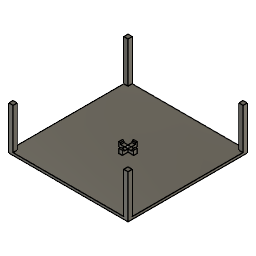
Desk (Autodesk Fusion 360 design; units mm, degrees)
part number: 2026-02-08-13-47-04-236
Autodesk Fusion 360 part; units mm, degrees
sketch "Sketch1" plane through (0, 0, 0) normal (0, 0, 1) x (1, 0, 0)
  line L0 (-44.8667, 47.2814) -> (95.1333, 47.2814)
  line L1 (95.1333, 47.2814) -> (95.1333, -92.7186)
  line L2 (95.1333, -92.7186) -> (-44.8667, -92.7186)
  line L3 (-44.8667, -92.7186) -> (-44.8667, 47.2814)
  dimension "d1" = 140
  dimension "d2" = 140
  constraint horizontal L0
  constraint vertical L1
  constraint horizontal L2
  constraint vertical L3
  measures "d1" distance of L0.start L0.end
  measures "d2" distance of L0.start L2.end
extrude "Extrude1" add sketch "Sketch1" along normal blind 3
sketch "Sketch2" plane through (0, 0, 3) normal (0, 0, 1) x (-1, 0, 0)
  line L0 (44.8667, 92.7186) -> (-95.1333, 92.7186)
  line L1 (-95.1333, 92.7186) -> (-95.1333, -47.2814)
  line L2 (-95.1333, -47.2814) -> (44.8667, -47.2814)
  line L3 (44.8667, -47.2814) -> (44.8667, 92.7186)
  line L4 (44.8667, -47.2814) -> (39.8667, -47.2814)
  line L5 (39.8667, -47.2814) -> (39.8667, -42.2814)
  line L6 (39.8667, -42.2814) -> (44.8667, -42.2814)
  line L7 (44.8667, -42.2814) -> (44.8667, -47.2814)
  line L8 (44.8667, 92.7186) -> (39.8667, 92.7186)
  line L9 (39.8667, 92.7186) -> (39.8667, 87.7186)
  line L10 (39.8667, 87.7186) -> (44.8667, 87.7186)
  line L11 (44.8667, 87.7186) -> (44.8667, 92.7186)
  line L12 (-95.1333, 92.7186) -> (-90.1333, 92.7186)
  line L13 (-90.1333, 92.7186) -> (-90.1333, 87.7186)
  line L14 (-90.1333, 87.7186) -> (-95.1333, 87.7186)
  line L15 (-95.1333, 87.7186) -> (-95.1333, 92.7186)
  line L16 (-95.1333, -47.2814) -> (-90.1333, -47.2814)
  line L17 (-90.1333, -47.2814) -> (-90.1333, -42.2814)
  line L18 (-90.1333, -42.2814) -> (-95.1333, -42.2814)
  line L19 (-95.1333, -42.2814) -> (-95.1333, -47.2814)
  dimension "d5" = 5
  dimension "d6" = 5
  dimension "d7" = 5
  dimension "d8" = 5
  dimension "d9" = 5
  dimension "d10" = 5
  dimension "d11" = 5
  dimension "d12" = 5
  constraint horizontal L4
  constraint vertical L5
  constraint horizontal L6
  constraint vertical L7
  constraint coincident L2.end L3.start
  constraint horizontal L8
  constraint vertical L9
  constraint horizontal L10
  constraint vertical L11
  constraint coincident L0.start L3.end
  constraint horizontal L12
  constraint vertical L13
  constraint horizontal L14
  constraint vertical L15
  constraint coincident L0.end L1.start
  constraint horizontal L16
  constraint vertical L17
  constraint horizontal L18
  constraint vertical L19
  constraint coincident L1.end L2.start
  measures "d5" distance of L2.end L4.end
  measures "d6" distance of L2.end L6.end
  measures "d7" distance of L0.start L8.end
  measures "d8" distance of L0.start L10.end
  measures "d9" distance of L0.end L12.end
  measures "d10" distance of L0.end L14.end
  measures "d11" distance of L1.end L16.end
  measures "d12" distance of L1.end L18.end
extrude "Extrude2" add sketch "Sketch2" along normal blind 48 contours L0 L3 L8 L9 L10 L11 | L0 L1 L12 L13 L14 L15 | L2 L3 L4 L5 L6 L7 | L1 L2 L16 L17 L18 L19
sketch "Sketch3" plane through (0, 0, 3) normal (0, 0, 1) x (-1, 0, 0)
  line L0 (-90.1333, 92.7186) -> (-90.1333, 87.7186)
  line L1 (-90.1333, 87.7186) -> (-95.1333, 87.7186)
  line L2 (-95.1333, 87.7186) -> (-95.1333, -42.2814)
  line L3 (-95.1333, -42.2814) -> (-90.1333, -42.2814)
  line L4 (-90.1333, -42.2814) -> (-90.1333, -47.2814)
  line L5 (-90.1333, -47.2814) -> (39.8667, -47.2814)
  line L6 (39.8667, -47.2814) -> (39.8667, -42.2814)
  line L7 (39.8667, -42.2814) -> (44.8667, -42.2814)
  line L8 (44.8667, -42.2814) -> (44.8667, 87.7186)
  line L9 (44.8667, 87.7186) -> (39.8667, 87.7186)
  line L10 (39.8667, 87.7186) -> (39.8667, 92.7186)
  line L11 (39.8667, 92.7186) -> (-90.1333, 92.7186)
  circle A0 centre (-25.1333, 22.7186) radius 2
  line L12 (-27.1333, 31.4686) -> (-23.1333, 31.4686)
  line L13 (-23.1333, 31.4686) -> (-23.1333, 13.9686)
  line L14 (-23.1333, 13.9686) -> (-27.1333, 13.9686)
  line L15 (-27.1333, 13.9686) -> (-27.1333, 31.4686)
  line L16 (-33.8833, 24.7186) -> (-16.3833, 24.7186)
  line L17 (-16.3833, 24.7186) -> (-16.3833, 20.7186)
  line L18 (-16.3833, 20.7186) -> (-33.8833, 20.7186)
  line L19 (-33.8833, 20.7186) -> (-33.8833, 24.7186)
  dimension "d15" = 4
  dimension "d16" = 70
  dimension "d17" = 70
  dimension "d18" = 4
  dimension "d19" = 17.5
  dimension "d20" = 8.75
  dimension "d21" = 2
  dimension "d22" = 17.5
  dimension "d23" = 4
  dimension "d24" = 2
  dimension "d25" = 8.75
  constraint horizontal L12
  constraint vertical L13
  constraint horizontal L14
  constraint vertical L15
  constraint horizontal L16
  constraint vertical L17
  constraint horizontal L18
  constraint vertical L19
  measures "d15" diameter of A0
  measures "d16" distance of L8 A0.centre
  measures "d17" distance of L11 A0.centre
  measures "d18" distance of L12.start L12.end
  measures "d19" distance of L12.start L14.end
  measures "d20" distance of A0.centre L12
  measures "d21" distance of A0.centre L15
  measures "d22" distance of L16.start L16.end
  measures "d23" distance of L16.start L18.end
  measures "d24" distance of A0.centre L18
  measures "d25" distance of A0.centre L19
extrude "Extrude3" add sketch "Sketch3" along normal blind 3.3 contours A0 L13 L18 | A0 L13 L16 | L13 L16 L17 L18 | A0 L15 L16 | L12 L13 L15 L16 | A0 L15 L18 | L13 L14 L15 L18 | L15 L16 L18 L19
sketch "Sketch4" plane through (0, 0, 6.3) normal (0, 0, 1) x (-1, 0, 0)
  circle A0 centre (-25.1333, 22.7186) radius 2
  line L0 (-33.8833, 20.7186) -> (-27.1333, 20.7186)
  line L1 (-27.1333, 20.7186) -> (-27.1333, 13.9686)
  line L2 (-27.1333, 13.9686) -> (-23.1333, 13.9686)
  line L3 (-23.1333, 13.9686) -> (-23.1333, 20.7186)
  line L4 (-23.1333, 20.7186) -> (-16.3833, 20.7186)
  line L5 (-16.3833, 20.7186) -> (-16.3833, 24.7186)
  line L6 (-16.3833, 24.7186) -> (-23.1333, 24.7186)
  line L7 (-23.1333, 24.7186) -> (-23.1333, 31.4686)
  line L8 (-23.1333, 31.4686) -> (-27.1333, 31.4686)
  line L9 (-27.1333, 31.4686) -> (-27.1333, 24.7186)
  line L10 (-27.1333, 24.7186) -> (-33.8833, 24.7186)
  line L11 (-33.8833, 24.7186) -> (-33.8833, 20.7186)
  line L12 (-27.1333, 31.4686) -> (-23.1333, 31.4686)
  line L13 (-23.1333, 31.4686) -> (-23.1333, 29.4686)
  line L14 (-23.1333, 29.4686) -> (-27.1333, 29.4686)
  line L15 (-27.1333, 29.4686) -> (-27.1333, 31.4686)
  line L16 (-16.3833, 24.7186) -> (-18.3833, 24.7186)
  line L17 (-18.3833, 24.7186) -> (-18.3833, 20.7186)
  line L18 (-18.3833, 20.7186) -> (-16.3833, 20.7186)
  line L19 (-16.3833, 20.7186) -> (-16.3833, 24.7186)
  line L20 (-23.1333, 13.9686) -> (-27.1333, 13.9686)
  line L21 (-27.1333, 13.9686) -> (-27.1333, 15.9686)
  line L22 (-27.1333, 15.9686) -> (-23.1333, 15.9686)
  line L23 (-23.1333, 15.9686) -> (-23.1333, 13.9686)
  line L24 (-33.8833, 24.7186) -> (-31.8833, 24.7186)
  line L25 (-31.8833, 24.7186) -> (-31.8833, 20.7186)
  line L26 (-31.8833, 20.7186) -> (-33.8833, 20.7186)
  line L27 (-33.8833, 20.7186) -> (-33.8833, 24.7186)
  dimension "d28" = 2
  dimension "d29" = 2
  dimension "d30" = 4
  dimension "d31" = 4
  dimension "d32" = 2
  dimension "d33" = 2
  dimension "d34" = 4
  dimension "d40" = 4
  constraint horizontal L12
  constraint vertical L13
  constraint horizontal L14
  constraint vertical L15
  constraint coincident L8.end L9.start
  constraint horizontal L16
  constraint vertical L17
  constraint horizontal L18
  constraint vertical L19
  constraint coincident L5.end L6.start
  constraint horizontal L20
  constraint vertical L21
  constraint horizontal L22
  constraint vertical L23
  constraint coincident L2.end L3.start
  constraint horizontal L24
  constraint vertical L25
  constraint horizontal L26
  constraint vertical L27
  constraint coincident L10.end L11.start
  measures "d28" distance of L8.end L14.end
  measures "d29" distance of L5.end L16.end
  measures "d30" distance of L5.end L4.end
  measures "d31" distance of L2.end L1.end
  measures "d32" distance of L2.end L22.end
  measures "d33" distance of L10.end L24.end
  measures "d34" distance of L10.end L0.start
  measures "d40" distance of L13.end L14.end
extrude "Extrude4" add sketch "Sketch4" along normal blind 2 contours L0 L10 L11 L24 L25 L26 L27 | L1 L2 L3 L20 L21 L22 L23 | L7 L8 L9 L12 L13 L14 L15 | L4 L5 L6 L16 L17 L18 L19
sketch "Sketch5" plane through (0, 0, 6.3) normal (0, 0, 1) x (-1, 0, 0)
  line L0 (-18.3833, 20.7186) -> (-18.3833, 24.7186)
  line L1 (-18.3833, 24.7186) -> (-23.1333, 24.7186)
  line L2 (-23.1333, 24.7186) -> (-23.1333, 29.4686)
  line L3 (-27.1333, 29.4686) -> (-27.1333, 24.7186)
  line L4 (-27.1333, 24.7186) -> (-31.8833, 24.7186)
  line L5 (-31.8833, 24.7186) -> (-31.8833, 20.7186)
  line L6 (-31.8833, 20.7186) -> (-27.1333, 20.7186)
  line L7 (-27.1333, 20.7186) -> (-27.1333, 15.9686)
  line L8 (-27.1333, 15.9686) -> (-23.1333, 15.9686)
  line L9 (-23.1333, 15.9686) -> (-23.1333, 20.7186)
  line L10 (-23.1333, 20.7186) -> (-18.3833, 20.7186)
  circle A0 centre (-25.1333, 22.7186) radius 2
  circle A1 centre (-25.1333, 22.7186) radius 16
  line L11 (-23.1333, 29.4686) -> (-27.1333, 29.4686)
  dimension "d37" = 32
  constraint concentric A0 A1
  measures "d37" diameter of A1
